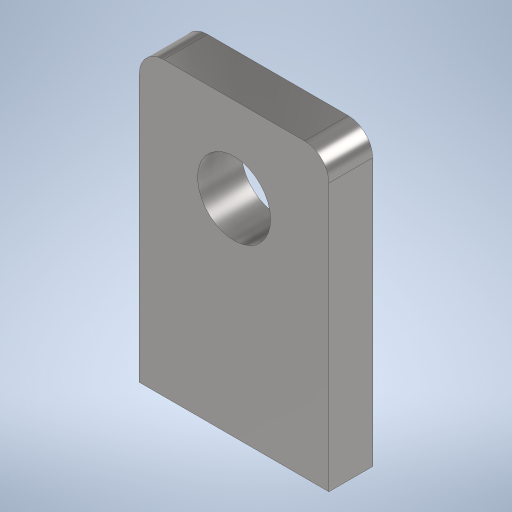
# Autodesk Inventor part: Limit switch pin
Saved by Autodesk Inventor 2023 (Build 270158000, 158)
## iProperties
Created: 2023-12-14
Part Number: Limit switch pin
Material: Stainless Steel
Document SubType Name: Modeling
Designer: User
Density: 8 g/cm^3
Appearance: Semi-Polished
Author: User
Autodesk Inventor part; units mm, degrees
ref_plane "YZ Plane" through (0, 0, 0) normal (1, 0, 0) x (0, 1, 0)
ref_plane "XZ Plane" through (0, 0, 0) normal (0, 1, 0) x (-1, 0, 0)
ref_plane "XY Plane" through (0, 0, 0) normal (0, 0, 1) x (1, 0, 0)
sketch "Sketch1" plane through (0, 0, 0) normal (0, 0, 1) x (1, 0, 0)
  line L0 (3.9, 0) -> (3.9, -6)
  line L1 (3.9, -6) -> (0, -6)
  line L2 (0, -6) -> (0, 0)
  line L3 (0.2186, 0) -> (3.3134, 0) construction
  line L4 (0.2186, -1) -> (3.3134, -1) construction
  line L5 (0.2186, -1.75) -> (3.3134, -1.75) construction
  line L6 (0, 1.467) -> (0, -3.9093) construction
  line L7 (1.95, 1.467) -> (1.95, -3.9093) construction
  circle A0 centre (1.95, -1.75) radius 0.75
  line L8 (0, 0) -> (3.9, 0)
  dimension "d0" = 3.9
  dimension "d1" = 6
  dimension "d2" = 1
  dimension "d3" = 0.75
  dimension "d4" = 1.95
  dimension "d5" = 1.5
  constraints: 18 end point, 4 parallel, 3 point on line, 1 centre point, 1 horizontal
  measures "d0" distance of L0.end L1.end
  measures "d1" distance of L0.start L0.end
  measures "d2" distance between parallel lines of L3 L4
  measures "d3" distance between parallel lines of L4 L5
  measures "d4" distance between parallel lines of L6 L7
  measures "d5" diameter of A0
extrude "Extrusion1" add sketch "Sketch1" along normal blind 0.9
fillet "Fillet1" radius 0.5 2 edges at (3.9, 0, 0.45) (0, 0, 0.45)
body "Solid1"
